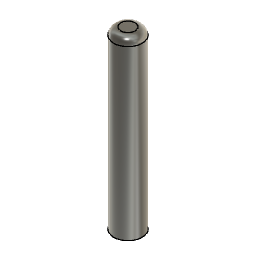
Pino Trava Porta Renault Kwid v1 (Autodesk Fusion 360 design; units mm, degrees)
Autodesk Fusion 360 part; units mm, degrees
sketch "Sketch1" plane through (0, 0, 0) normal (0, 0, 1) x (1, 0, 0)
  circle A0 centre (40, 20) radius 2
  circle A1 centre (40, 20) radius 4
  dimension "d1" = 4
  dimension "d2" = 8
  constraint concentric A0 A1
  measures "d1" diameter of A0
  measures "d2" diameter of A1
extrude "Extrude1" add sketch "Sketch1" along normal blind 35 makes body 1
sketch "Sketch2" plane through (0, 0, 35) normal (0, 0, 1) x (-1, 0, 0)
  circle A0 centre (-40, -20) radius 2
  circle A1 centre (-40, -20) radius 4
  circle A2 centre (-40, -20) radius 4
  circle A3 centre (-40, -20) radius 2
  dimension "d5" = 8
  constraint concentric A2 A3
  measures "d5" diameter of A2
extrude "Extrude2" add sketch "Sketch2" along normal blind 14.3 separate body contours A0 A3 makes body 2
extrude "Extrude3" add 1 faces at (43.311, 19.7019, 35) along direction (0, 0, 1) blind 14.3 on bodies 1 bodies 1 2
fillet "Fillet1" radius 2 1 edges at (36.2707, 18.5535, 49.3) on bodies 1
